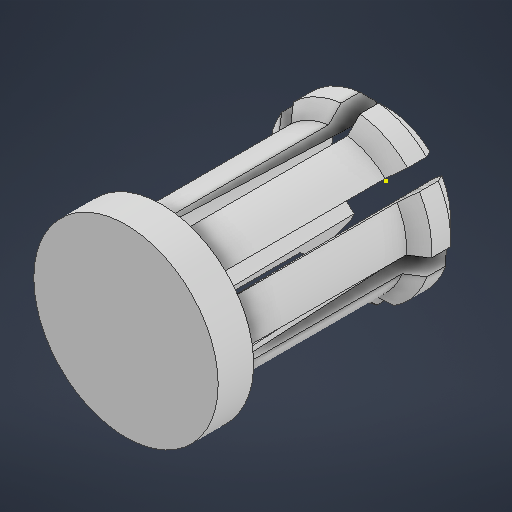
# Autodesk Inventor part: WirePlugs
Saved by Autodesk Inventor 2026.2 (Build 302298000, 298)
## iProperties
Created: 2026-05-27
Part Number: WirePlugs
Material: Generic
Document SubType Name: Modeling
Designer: mayhe
Density: 1 g/cm^3
Appearance: Default
Author: mayhe
Autodesk Inventor part; units mm, degrees
ref_plane "YZ Plane" through (0, 0, 0) normal (1, 0, 0) x (0, 1, 0)
ref_plane "XZ Plane" through (0, 0, 0) normal (0, 1, 0) x (-1, 0, 0)
ref_plane "XY Plane" through (0, 0, 0) normal (0, 0, 1) x (1, 0, 0)
sketch "Sketch1" plane through (0, 0, 0) normal (0, 0, 1) x (1, 0, 0)
  circle A0 centre (0, 0) radius 19.5
  dimension "d0" = 39
  constraints: 1 centre point, 1 coincident
  measures "d0" diameter of A0
extrude "Body" add sketch "Sketch1" along normal mid plane 55
sketch "Sketch2" plane through (0, 0, -27.5) normal (0, 0, -1) x (-1, 0, 0)
  point P0 (0, 0)
sketch "Sketch3" plane through (0, 0, 0) normal (1, 0, 0) x (0, 1, 0)
  line L0 (19.5, 20) -> (14.5, 20)
  line L1 (14.5, 20) -> (14.5, -20)
  line L2 (14.5, -20) -> (17.15, -20)
  line L3 (17.15, -20) -> (17.15, -27.5)
  line L4 (-19.5, -27.5) -> (19.5, -27.5) projected
  line L5 (19.5, 20) -> (19.5, -27.5)
  line L6 (17.15, -27.5) -> (19.5, -27.5)
  line L7 (0, -38.5) -> (0, 38.5) projected
  line L8 (19.5, 27.5) -> (-19.5, 27.5) projected
  point P0 (0, 0)
  dimension "d4" = 5
  dimension "d5" = 40
  dimension "d6" = 2.65
  dimension "d27" = 7.5
  constraints: 12 end point, 3 perpendicular, 1 collinear, 1 horizontal, 1 point on line
  measures "d4" distance of L0.start L0.end
  measures "d5" distance of L0.end L1.end
  measures "d6" distance of L1.end L2.end
  measures "d27" distance from line of L8 L0.start
revolve "Revolution1" cut sketch "Sketch3" angle 360 about axis through (0, 0, -10) along (0, 0, 1)
chamfer "Chamfer1" distance 3.5 angle 45 1 edges at (0, -17.15, -27.5)
chamfer "Chamfer2" distance 2.65 angle 45 1 edges at (0, -14.5, -20)
sketch "Sketch4" plane through (0, 0, -27.5) normal (0, 0, -1) x (-1, 0, 0)
  circle A0 centre (0, 0) radius 11.5
  dimension "d14" = 23
  constraints: 1 centre point, 1 coincident
  measures "d14" diameter of A0
extrude "Extrusion2" cut sketch "Sketch4" against normal up to surface (47.5 mm away) draft 2.5
sketch "Sketch5" plane through (0, 0, -27.5) normal (0, 0, -1) x (-1, 0, 0)
  line L0 (-2, 18.114) -> (2, 18.114)
  line L1 (2, 18.114) -> (2, 9.186)
  line L2 (2, 9.186) -> (-2, 9.186)
  line L3 (-2, 9.186) -> (-2, 18.114)
  circle A0 centre (0, 0) radius 13.65 projected
  line L4 (-2, 18.114) -> (2, 9.186) construction
  line L5 (2, 18.114) -> (-2, 9.186) construction
  line L6 (-15.4091, 9.7302) -> (-12.9151, 12.8576)
  line L7 (-12.9151, 12.8576) -> (-8.4289, 4.1637) construction
  line L8 (-12.9151, 12.8576) -> (-5.9349, 7.291)
  line L9 (-15.4091, 9.7302) -> (-5.9349, 7.291) construction
  line L10 (-8.4289, 4.1637) -> (-15.4091, 9.7302)
  line L11 (-5.9349, 7.291) -> (-8.4289, 4.1637)
  line L12 (-17.2148, -5.9806) -> (-18.1049, -2.0809)
  line L13 (-18.1049, -2.0809) -> (-8.5106, -3.9939) construction
  line L14 (-18.1049, -2.0809) -> (-9.4007, -0.0942)
  line L15 (-17.2148, -5.9806) -> (-9.4007, -0.0942) construction
  line L16 (-8.5106, -3.9939) -> (-17.2148, -5.9806)
  line L17 (-9.4007, -0.0942) -> (-8.5106, -3.9939)
  line L18 (-6.0574, -17.1879) -> (-9.6613, -15.4524)
  line L19 (-9.6613, -15.4524) -> (-2.1837, -9.144) construction
  line L20 (-9.6613, -15.4524) -> (-5.7876, -7.4085)
  line L21 (-6.0574, -17.1879) -> (-5.7876, -7.4085) construction
  line L22 (-2.1837, -9.144) -> (-6.0574, -17.1879)
  line L23 (-5.7876, -7.4085) -> (-2.1837, -9.144)
  line L24 (9.6613, -15.4524) -> (6.0574, -17.1879)
  line L25 (6.0574, -17.1879) -> (5.7876, -7.4085) construction
  line L26 (6.0574, -17.1879) -> (2.1837, -9.144)
  line L27 (9.6613, -15.4524) -> (2.1837, -9.144) construction
  line L28 (5.7876, -7.4085) -> (9.6613, -15.4524)
  line L29 (2.1837, -9.144) -> (5.7876, -7.4085)
  line L30 (18.1049, -2.0809) -> (17.2148, -5.9806)
  line L31 (17.2148, -5.9806) -> (9.4007, -0.0942) construction
  line L32 (17.2148, -5.9806) -> (8.5106, -3.9939)
  line L33 (18.1049, -2.0809) -> (8.5106, -3.9939) construction
  line L34 (9.4007, -0.0942) -> (18.1049, -2.0809)
  line L35 (8.5106, -3.9939) -> (9.4007, -0.0942)
  line L36 (12.9151, 12.8576) -> (15.4091, 9.7302)
  line L37 (15.4091, 9.7302) -> (5.9349, 7.291) construction
  line L38 (15.4091, 9.7302) -> (8.4289, 4.1637)
  line L39 (12.9151, 12.8576) -> (8.4289, 4.1637) construction
  line L40 (5.9349, 7.291) -> (12.9151, 12.8576)
  line L41 (8.4289, 4.1637) -> (5.9349, 7.291)
  point P0 (0, 13.65)
  point P1 (-10.672, 8.5106)
  point P2 (-13.3078, -3.0374)
  point P3 (-5.9225, -12.2982)
  point P4 (5.9225, -12.2982)
  point P5 (13.3078, -3.0374)
  point P6 (10.672, 8.5106)
  dimension "d17" = 4
  dimension "d20" = 360
  constraints: 84 end point, 2 midpoint, 2 parallel, 1 horizontal, 1 perpendicular, 1 vertical alignment, 79 other
  measures "d17" distance of L1.end L2.end
extrude "Extrusion3" cut sketch "Sketch5" against normal up to surface (47.5 mm away) contours L0 L1 A0 L3 | A0 L1 L2 L3 | L8 L11 L10 A0 | A0 L10 L6 L8 | L40 L36 L38 A0 | A0 L38 L41 L40 | L14 L17 L16 A0 | A0 L16 L12 L14 | L34 L30 L32 A0 | A0 L32 L35 L34 | L20 L23 L22 A0 | A0 L22 L18 L20 | L28 L24 L26 A0 | A0 L26 L29 L28
chamfer "Chamfer3" distance 1 angle 45 14 edges at (-2, 13.8936, 20) (2, 13.8936, 20) (9.6155, 10.2262, 20) (12.1094, 7.0988, 20) (13.9903, -1.1418, 20) (13.1002, -5.0415, 20) (7.8301, -11.6499, 20) (4.2263, -13.3854, 20) (-4.2263, -13.3854, 20) (-7.8301, -11.6499, 20) (-13.1002, -5.0415, 20) (-13.9903, -1.1418, 20) (-12.1094, 7.0988, 20) (-9.6155, 10.2262, 20)
body "Solid1"
